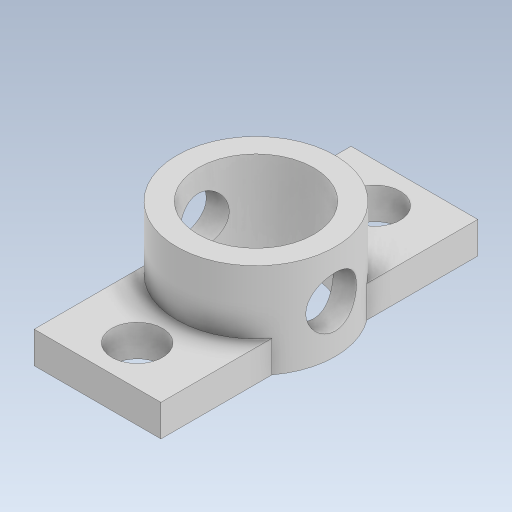
# Autodesk Inventor part: Fix Bracket Lifter
Saved by Autodesk Inventor 2023.5 (Build 275446000, 446)
## iProperties
Created: 2025-10-01
Part Number: Fix Bracket Lifter
Material: Generic
Document SubType Name: Modeling
Designer: Guntur
Density: 1 g/cm^3
Appearance: Default
Author: Guntur
Autodesk Inventor part; units mm, degrees
ref_plane "YZ Plane" through (0, 0, 0) normal (1, 0, 0) x (0, 1, 0)
ref_plane "XZ Plane" through (0, 0, 0) normal (0, 1, 0) x (-1, 0, 0)
ref_plane "XY Plane" through (0, 0, 0) normal (0, 0, 1) x (1, 0, 0)
sketch "Sketch1" plane through (0, 0, 0) normal (0, 1, 0) x (-1, 0, 0)
  circle A0 centre (0, 0) radius 3.65
  circle A1 centre (0, 0) radius 5
  line L0 (4, 10) -> (-4, 10)
  line L1 (-4, 10) -> (-4, -10)
  line L2 (-4, -10) -> (4, -10)
  line L3 (4, -10) -> (4, 10)
  line L4 (4, 10) -> (-4, -10) construction
  line L5 (-4, 10) -> (4, -10) construction
  circle A2 centre (0, 7.5) radius 1.6
  circle A3 centre (0, -7.5) radius 1.6
  point P0 (4, -3)
  point P1 (-4, -3)
  point P2 (4, 3)
  point P3 (-4, 3)
  dimension "d0" = 7.3
  dimension "d1" = 10
  dimension "d2" = 20
  dimension "d3" = 3.2
  dimension "d4" = 2.5
  dimension "d5" = 3.2
  dimension "d6" = 2.5
  constraints: 12 end point, 4 centre point, 2 coincident, 2 midpoint, 2 parallel, 1 horizontal, 1 perpendicular
  measures "d0" diameter of A0
  measures "d1" diameter of A1
  measures "d2" distance of L1.end L0.end
  measures "d3" diameter of A2
  measures "d4" distance from line of L0 A2.centre
  measures "d5" diameter of A3
  measures "d6" distance from line of L2 A3.centre
extrude "Extrusion1" add sketch "Sketch1" along normal blind 2 contours A1 L3 | A1 L1 L0 L3 | L3 L2 L1 A1 | L1 A1
extrude "Extrusion2" add sketch "Sketch1" along normal blind 6 contours A1 L3 | L3 A1 L1 | L1 A1
ref_plane "Work Plane1" through (5, 0, 0) normal (1, 0, 0) x (0, 0, -1)
sketch "Sketch2" plane through (5, 0, 0) normal (1, 0, 0) x (0, 0, -1)
  circle A0 centre (0, 3) radius 1.6
  point P0 (0, 0)
  dimension "d11" = 3.2
  constraints: 1 centre point
  measures "d11" diameter of A0
extrude "Extrusion3" cut sketch "Sketch2" against normal blind 10
body "Solid1"
